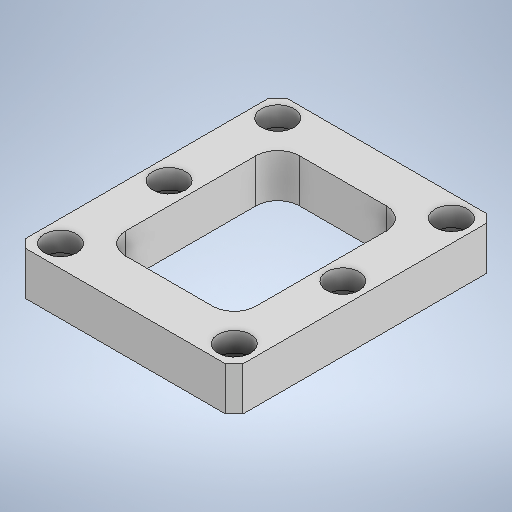
# Autodesk Inventor part: peca3
Saved by Autodesk Inventor 2025.1 (Build 291241000, 241)
## iProperties
Created: 2024-08-25
Part Number: peca3
Material: Generic
Document SubType Name: Modeling
Designer: pedro
Density: 1 g/cm^3
Appearance: Default
Author: pedro
Autodesk Inventor part; units mm, degrees
ref_plane "YZ Plane" through (0, 0, 0) normal (1, 0, 0) x (0, 1, 0)
ref_plane "XZ Plane" through (0, 0, 0) normal (0, 1, 0) x (-1, 0, 0)
ref_plane "XY Plane" through (0, 0, 0) normal (0, 0, 1) x (1, 0, 0)
sketch "Sketch1" plane through (0, 0, 0) normal (0, 1, 0) x (-1, 0, 0)
  line L0 (-50, 60) -> (50, 60)
  line L1 (50, 60) -> (50, -60)
  line L2 (50, -60) -> (-50, -60)
  line L3 (-50, -60) -> (-50, 60)
  line L4 (-50, 60) -> (50, -60) construction
  line L5 (50, 60) -> (-50, -60) construction
  line L6 (30, 40) -> (-30, 40)
  line L7 (-30, 40) -> (-30, -40)
  line L8 (-30, -40) -> (30, -40)
  line L9 (30, -40) -> (30, 40)
  line L10 (30, 40) -> (-30, -40) construction
  line L11 (-30, 40) -> (30, -40) construction
  point P0 (0, 0)
  dimension "d0" = 100
  dimension "d1" = 120
  dimension "d2" = 60
  dimension "d3" = 80
  constraints: 24 end point, 4 midpoint, 4 parallel, 2 horizontal, 2 perpendicular
  measures "d0" distance of L1.end L2.end
  measures "d1" distance of L0.end L1.end
  measures "d2" distance of L8.end L7.end
  measures "d3" distance of L7.end L6.end
extrude "Extrusion1" add sketch "Sketch1" along normal blind 20
sketch "Sketch2" plane through (0, 20, 0) normal (0, 1, 0) x (1, 0, 0)
  circle A0 centre (-40, 50) radius 4.5
  line L0 (-50, 60) -> (-50, -60) projected
  circle A1 centre (-40, 0) radius 4.5
  circle A2 centre (-40, -50) radius 4.5
  line L1 (0, -4.5) -> (0, 7.1494) construction
  circle A3 centre (40, 50) radius 4.5
  circle A4 centre (40, 0) radius 4.5
  circle A5 centre (40, -50) radius 4.5
  point P0 (0, 0)
  dimension "d6" = 9
  dimension "d7" = 10
  dimension "d8" = 50
  dimension "d9" = 9
  dimension "d10" = 9
  dimension "d11" = 50
  constraints: 6 centre point, 3 symmetric about line, 2 end point, 1 vertical, 3 other
  measures "d6" diameter of A0
  measures "d7" distance from line of L0 A0.centre
  measures "d8" vertical distance of point (0, 0) A0.centre
  measures "d9" diameter of A1
  measures "d10" diameter of A2
  measures "d11" vertical distance of A2.centre point (0, 0)
extrude "Extrusion2" cut sketch "Sketch2" against normal through all
sketch "Sketch3" plane through (0, 20, 0) normal (0, 1, 0) x (1, 0, 0)
  circle A0 centre (-40, 50) radius 4.5 projected
  circle A1 centre (-40, 50) radius 7.5
  circle A2 centre (-40, 0) radius 4.5 projected
  circle A3 centre (-40, 0) radius 7.5
  circle A4 centre (-40, -50) radius 4.5 projected
  circle A5 centre (-40, -50) radius 7.5
  circle A6 centre (40, -50) radius 4.5 projected
  circle A7 centre (40, -50) radius 7.5
  circle A8 centre (40, 0) radius 4.5 projected
  circle A9 centre (40, 0) radius 7.5
  circle A10 centre (40, 50) radius 4.5 projected
  circle A11 centre (40, 50) radius 7.5
  point P0 (0, 0)
  dimension "d14" = 15
  dimension "d15" = 15
  dimension "d16" = 15
  dimension "d17" = 15
  dimension "d18" = 15
  dimension "d19" = 15
  constraints: 6 centre point, 6 coincident
  measures "d14" diameter of A1
  measures "d15" diameter of A3
  measures "d16" diameter of A5
  measures "d17" diameter of A7
  measures "d18" diameter of A9
  measures "d19" diameter of A11
extrude "Extrusion3" cut sketch "Sketch3" against normal blind 9
fillet "Fillet1" radius 10 4 edges at (-30, 10, -40) (-30, 10, 40) (30, 10, 40) (30, 10, -40)
chamfer "Chamfer1" distance 4 angle 45 4 edges at (50, 10, 60) (-50, 10, 60) (-50, 10, -60) (50, 10, -60)
body "Solid1"
